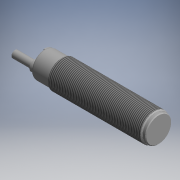
# Autodesk Inventor part: BALLUFF BCS M18BBN1-PSC80D-EP021
Saved by Autodesk Inventor 2017.3 (Build 213256000, 256)
## iProperties
Part Number: BALLUFF BCS M18BBN1-PSC80D-EP021
Material: Generic
Catalog Web Link: www.cadenas.de
Description: BCS M18 x 1-1-
Vendor: BALLUFF
Document SubType Name: Modeling
Designer: partserver
Manufacturer: BALLUFF
Mass: 18.277 g
Surface Area: 47.7442 cm^2
Volume: 18.277 cm^3
Density: 1 g/cm^3
Appearance: PSOLRGB-192-192-192
Category: PARTsolutions
Company: BALLUFF
Title: BALLUFF BCS M18BBN1-PSC80D-EP021
Author: Cadenas PARTsolutions
PSOL_IDENT_0: {$CADENAS_DATA\23d-libs\balluff\sensortechnik\kapazitive\bcs_18.prj},213 {VTYP=3D},{NB=BALLUFF BCS M
PSOL_IDENT_1: 18BBN1-PSC80D-EP021},{LINA=BALLUFF BCS M18BBN1-PSC80D-EP021},{NN=BCS M18 x 1-1},{DATE=15.02.2021 22:
PSOL_IDENT_2: 54:46},{GEOMDATE=02.12.2020 12:07:00},{VERSION=},{LINEID=1410},{WBVAR=},{WBNUMERIC=}  {NB=BALLUFF BC
PSOL_IDENT_3: S M18BBN1-PSC80D-EP021},{LINA=BALLUFF BCS M18BBN1-PSC80D-EP021},{KT=DUMMY},{BC=BCS00NZ},{AB=BCS M18B
PSOL_IDENT_4: BN1-PSC80D-EP02},{AB1=BCS_M18BBN1-PSC80D-EP02},{PX=45636_00},{PXX=45636},{LM1=22.000},{LM2=31.000}
NB: BALLUFF BCS M18BBN1-PSC80D-EP021
NN: BCS M18 x 1-1
NBSYN: BALLUFF $AB.1
LINA: BALLUFF BCS M18BBN1-PSC80D-EP021
CATALOG: Balluff
BC: BCS00NZ
AB: BCS M18BBN1-PSC80D-EP02
AB1: BCS_M18BBN1-PSC80D-EP02
PX: 45636_00
PXX: 45636
LM1: 22
LM2: 31
SUPPLIER: BALLUFF
ARTICLENO: BALLUFF BCS M18BBN1-PSC80D-EP021
BOMINFO: BALLUFF BCS M18BBN1-PSC80D-EP021
CREATOR: CADENAS GmbH
Autodesk Inventor part; units mm, degrees
sketch "Sketch_1" plane through (0, 0, 0) normal (0, 0, 1) x (1, 0, 0)
  line L0 (60, 0) -> (-12.5, 0)
  line L1 (-12.5, 0) -> (-12.5, 7.8757)
  line L2 (-12.5, 7.8757) -> (-12.0757, 8.3)
  line L3 (-12.0757, 8.3) -> (-10.5, 8.3)
  line L4 (-10.5, 8.3) -> (-10.5, 8.3865)
  line L5 (-10.5, 8.3865) -> (-9.8865, 9)
  line L6 (-9.8865, 9) -> (48.8865, 9)
  line L7 (48.8865, 9) -> (49.5, 8.3865)
  line L8 (49.5, 8.3865) -> (49.5, 8.3)
  line L9 (49.5, 8.3) -> (58.97, 8.3)
  line L10 (58.97, 8.3) -> (58.97, 8.15)
  line L11 (58.97, 8.15) -> (59.5, 8.15)
  line L12 (59.5, 8.15) -> (60, 8.05)
  line L13 (60, 8.05) -> (60, 0)
  line L14 (60, 0) -> (-12.5, 0)
  constraints: 30 end point
revolve "Revolution1" add sketch "Sketch_1" angle 360 about axis through (60, 0, 0) along (1, 0, 0)
thread "Thread1" size "M18x1" class "6g" standard "ISO Metric profile" full length
sketch "Sketch_2" plane through (0, 0, 0) normal (0, 0, 1) x (1, 0, 0)
  line L0 (75, -4) -> (60, -4)
  line L1 (60, -4) -> (60, -0.65)
  line L2 (60, -0.65) -> (62.5, -0.65)
  line L3 (62.5, -0.65) -> (62.5, -1.75)
  line L4 (62.5, -1.75) -> (75, -1.75)
  line L5 (75, -1.75) -> (75, -4)
  line L6 (75, -4) -> (60, -4)
  constraints: 14 end point
revolve "Revolution2" add sketch "Sketch_2" angle 360 about axis through (75, -4, 0) along (1, 0, 0)
sketch "Sketch_5" plane through (60.7, 0, 0) normal (1, 0, 0) x (0, 0, -1)
  line L0 (1.4, 7.8765) -> (1.4, 0)
  line L1 (1.4, 0) -> (7.6942, 0)
  arc A0 (7.6942, 0) -> (7.9939, 0.3117) centre (7.6942, 0.3) ccw
  arc A1 (7.9939, 0.3117) -> (1.4, 7.8765) centre (0, 0) ccw
  constraints: 4 end point, 4 point on circle, 2 centre point
extrude "Extrusion1" add sketch "Sketch_5" against normal blind 0.7
sketch "Sketch_9" plane through (60.7, 0, 0) normal (1, 0, 0) x (0, 0, -1)
  arc A0 (-7.9822, 0.5333) -> (-7.4833, 0) centre (-7.4833, 0.5) ccw
  line L0 (-7.4833, 0) -> (-1.4026, 0)
  line L1 (-1.4026, 0) -> (-1.4026, 7.8761)
  arc A1 (-1.4026, 7.8761) -> (-7.9822, 0.5333) centre (0, 0) ccw
  constraints: 4 end point, 4 point on circle, 2 centre point
extrude "Extrusion2" add sketch "Sketch_9" against normal blind 0.7
sketch "Sketch_10" plane through (60.7, 0, 0) normal (1, 0, 0) x (0, 0, -1)
  circle A0 centre (0, 1.4) radius 1.4
  constraints: 1 centre point
extrude "Extrusion3" cut sketch "Sketch_10" against normal blind 1.5
sketch "Sketch_6" plane through (60.7, 0, 0) normal (1, 0, 0) x (0, 0, -1)
  line L0 (-0.25, 0) -> (0.25, 0)
  line L1 (0.25, 0) -> (0.25, 2.8)
  line L2 (0.25, 2.8) -> (-0.25, 2.8)
  line L3 (-0.25, 2.8) -> (-0.25, 0)
  constraints: 8 end point
extrude "Extrusion4" add sketch "Sketch_6" against normal blind 1.1
ref_plane "ip1_XY" through (0, 0, 0) normal (1, 0, 0) x (0, 0, -1)
ref_plane "ip1_YZ" through (0, 0, 0) normal (0, 0, -1) x (0, 1, 0)
ref_plane "ip1_ZX" through (0, 0, 0) normal (0, 1, 0) x (1, 0, 0)
body "Solid1"
